Autodesk Inventor part; units mm, degrees
(part 7 of 13)
  arc A2356 (6.9015, 50.997) -> (6.9497, 50.8806) centre (6.9256, 50.9388) ccw
  line L2355 (6.9497, 50.8806) -> (7.4521, 51.0887)
  arc A2357 (7.4521, 51.0887) -> (7.4039, 51.2051) centre (7.428, 51.1469) ccw
  line L2356 (6.8811, 50.9833) -> (6.4966, 50.5988)
  arc A2358 (6.4966, 50.5988) -> (6.5856, 50.5098) centre (6.5411, 50.5543) ccw
  line L2357 (6.5856, 50.5098) -> (6.9701, 50.8943)
  arc A2359 (6.9701, 50.8943) -> (6.8811, 50.9833) centre (6.9256, 50.9388) ccw
  line L2358 (6.4829, 50.5784) -> (6.2748, 50.076)
  arc A2360 (6.2748, 50.076) -> (6.3912, 50.0278) centre (6.333, 50.0519) ccw
  line L2359 (6.3912, 50.0278) -> (6.5993, 50.5302)
  arc A2361 (6.5993, 50.5302) -> (6.4829, 50.5784) centre (6.5411, 50.5543) ccw
  line L2360 (6.27, 50.0519) -> (6.27, 49.8428)
  arc A2362 (6.27, 49.8428) -> (6.396, 49.8428) centre (6.333, 49.8428) ccw
  line L2361 (6.396, 49.8428) -> (6.396, 50.0519)
  arc A2363 (6.396, 50.0519) -> (6.27, 50.0519) centre (6.333, 50.0519) ccw
  line L2362 (6.333, 49.7798) -> (7.6365, 49.7798)
  arc A2364 (7.6365, 49.7798) -> (7.6365, 49.9058) centre (7.6365, 49.8428) ccw
  line L2363 (7.6365, 49.9058) -> (6.333, 49.9058)
  arc A2365 (6.333, 49.9058) -> (6.333, 49.7798) centre (6.333, 49.8428) ccw
  line L2364 (7.5735, 49.8428) -> (7.5735, 49.717)
  arc A2366 (7.5735, 49.717) -> (7.6995, 49.717) centre (7.6365, 49.717) ccw
  line L2365 (7.6995, 49.717) -> (7.6995, 49.8428)
  arc A2367 (7.6995, 49.8428) -> (7.5735, 49.8428) centre (7.6365, 49.8428) ccw
  line L2366 (7.6365, 49.78) -> (6.333, 49.78)
  arc A2368 (6.333, 49.78) -> (6.333, 49.654) centre (6.333, 49.717) ccw
  line L2367 (6.333, 49.654) -> (7.6365, 49.654)
  arc A2369 (7.6365, 49.654) -> (7.6365, 49.78) centre (7.6365, 49.717) ccw
  line L2368 (6.27, 49.717) -> (6.27, 49.508)
  arc A2370 (6.27, 49.508) -> (6.396, 49.508) centre (6.333, 49.508) ccw
  line L2369 (6.396, 49.508) -> (6.396, 49.717)
  arc A2371 (6.396, 49.717) -> (6.27, 49.717) centre (6.333, 49.717) ccw
  line L2370 (6.2748, 49.4839) -> (6.4829, 48.9815)
  arc A2372 (6.4829, 48.9815) -> (6.5993, 49.0297) centre (6.5411, 49.0056) ccw
  line L2371 (6.5993, 49.0297) -> (6.3912, 49.5321)
  arc A2373 (6.3912, 49.5321) -> (6.2748, 49.4839) centre (6.333, 49.508) ccw
  line L2372 (6.4966, 48.9611) -> (6.8811, 48.5766)
  arc A2374 (6.8811, 48.5766) -> (6.9701, 48.6656) centre (6.9256, 48.6211) ccw
  line L2373 (6.9701, 48.6656) -> (6.5856, 49.0501)
  arc A2375 (6.5856, 49.0501) -> (6.4966, 48.9611) centre (6.5411, 49.0056) ccw
  line L2374 (6.9015, 48.5629) -> (7.4039, 48.3548)
  arc A2376 (7.4039, 48.3548) -> (7.4521, 48.4712) centre (7.428, 48.413) ccw
  line L2375 (7.4521, 48.4712) -> (6.9497, 48.6793)
  arc A2377 (6.9497, 48.6793) -> (6.9015, 48.5629) centre (6.9256, 48.6211) ccw
  line L2376 (1.0789, 1.071) -> (17.121, 1.071)
  arc A2378 (17.121, 1.071) -> (17.121, 1.197) centre (17.121, 1.134) ccw
  line L2377 (17.121, 1.197) -> (1.0789, 1.197)
  arc A2379 (1.0789, 1.197) -> (1.0789, 1.071) centre (1.0789, 1.134) ccw
  line L2378 (1.0789, 1.197) -> (17.121, 1.197)
  arc A2380 (17.121, 1.197) -> (17.121, 1.323) centre (17.121, 1.26) ccw
  line L2379 (17.121, 1.323) -> (1.0789, 1.323)
  arc A2381 (1.0789, 1.323) -> (1.0789, 1.197) centre (1.0789, 1.26) ccw
  line L2380 (1.0789, 1.323) -> (17.121, 1.323)
  arc A2382 (17.121, 1.323) -> (17.121, 1.449) centre (17.121, 1.386) ccw
  line L2381 (17.121, 1.449) -> (1.0789, 1.449)
  arc A2383 (1.0789, 1.449) -> (1.0789, 1.323) centre (1.0789, 1.386) ccw
  line L2382 (1.0789, 1.449) -> (17.121, 1.449)
  arc A2384 (17.121, 1.449) -> (17.121, 1.575) centre (17.121, 1.512) ccw
  line L2383 (17.121, 1.575) -> (1.0789, 1.575)
  arc A2385 (1.0789, 1.575) -> (1.0789, 1.449) centre (1.0789, 1.512) ccw
  line L2384 (1.0789, 1.575) -> (17.121, 1.575)
  arc A2386 (17.121, 1.575) -> (17.121, 1.701) centre (17.121, 1.638) ccw
  line L2385 (17.121, 1.701) -> (1.0789, 1.701)
  arc A2387 (1.0789, 1.701) -> (1.0789, 1.575) centre (1.0789, 1.638) ccw
  line L2386 (1.0789, 1.701) -> (17.121, 1.701)
  arc A2388 (17.121, 1.701) -> (17.121, 1.827) centre (17.121, 1.764) ccw
  line L2387 (17.121, 1.827) -> (1.0789, 1.827)
  arc A2389 (1.0789, 1.827) -> (1.0789, 1.701) centre (1.0789, 1.764) ccw
  line L2388 (1.0789, 1.827) -> (17.121, 1.827)
  arc A2390 (17.121, 1.827) -> (17.121, 1.953) centre (17.121, 1.89) ccw
  line L2389 (17.121, 1.953) -> (1.0789, 1.953)
  arc A2391 (1.0789, 1.953) -> (1.0789, 1.827) centre (1.0789, 1.89) ccw
  line L2390 (1.0789, 1.953) -> (17.121, 1.953)
  arc A2392 (17.121, 1.953) -> (17.121, 2.079) centre (17.121, 2.016) ccw
  line L2391 (17.121, 2.079) -> (1.0789, 2.079)
  arc A2393 (1.0789, 2.079) -> (1.0789, 1.953) centre (1.0789, 2.016) ccw
  line L2392 (1.0789, 2.079) -> (17.121, 2.079)
  arc A2394 (17.121, 2.079) -> (17.121, 2.205) centre (17.121, 2.142) ccw
  line L2393 (17.121, 2.205) -> (1.0789, 2.205)
  arc A2395 (1.0789, 2.205) -> (1.0789, 2.079) centre (1.0789, 2.142) ccw
  line L2394 (1.0789, 2.205) -> (17.121, 2.205)
  arc A2396 (17.121, 2.205) -> (17.121, 2.331) centre (17.121, 2.268) ccw
  line L2395 (17.121, 2.331) -> (1.0789, 2.331)
  arc A2397 (1.0789, 2.331) -> (1.0789, 2.205) centre (1.0789, 2.268) ccw
  line L2396 (1.0789, 2.331) -> (17.121, 2.331)
  arc A2398 (17.121, 2.331) -> (17.121, 2.457) centre (17.121, 2.394) ccw
  line L2397 (17.121, 2.457) -> (1.0789, 2.457)
  arc A2399 (1.0789, 2.457) -> (1.0789, 2.331) centre (1.0789, 2.394) ccw
  line L2398 (1.0789, 2.457) -> (17.121, 2.457)
  arc A2400 (17.121, 2.457) -> (17.121, 2.583) centre (17.121, 2.52) ccw
  line L2399 (17.121, 2.583) -> (1.0789, 2.583)
  arc A2401 (1.0789, 2.583) -> (1.0789, 2.457) centre (1.0789, 2.52) ccw
  line L2400 (1.0789, 2.583) -> (17.121, 2.583)
  arc A2402 (17.121, 2.583) -> (17.121, 2.709) centre (17.121, 2.646) ccw
  line L2401 (17.121, 2.709) -> (1.0789, 2.709)
  arc A2403 (1.0789, 2.709) -> (1.0789, 2.583) centre (1.0789, 2.646) ccw
  line L2402 (1.0789, 2.709) -> (17.121, 2.709)
  arc A2404 (17.121, 2.709) -> (17.121, 2.835) centre (17.121, 2.772) ccw
  line L2403 (17.121, 2.835) -> (1.0789, 2.835)
  arc A2405 (1.0789, 2.835) -> (1.0789, 2.709) centre (1.0789, 2.772) ccw
  line L2404 (1.0789, 2.835) -> (6.4573, 2.835)
  arc A2406 (6.4573, 2.835) -> (6.4573, 2.961) centre (6.4573, 2.898) ccw
  line L2405 (6.4573, 2.961) -> (1.0789, 2.961)
  arc A2407 (1.0789, 2.961) -> (1.0789, 2.835) centre (1.0789, 2.898) ccw
  line L2406 (8.9426, 2.835) -> (17.121, 2.835)
  line L2407 (1.0789, 49.833) -> (1.7644, 49.833)
  line L2408 (17.121, 2.961) -> (8.9426, 2.961)
  arc A2408 (8.9426, 2.961) -> (8.9426, 2.835) centre (8.9426, 2.898) ccw
  line L2409 (1.0789, 2.961) -> (6.4346, 2.961)
  arc A2409 (6.4346, 2.961) -> (6.4346, 3.087) centre (6.4346, 3.024) ccw
  line L2410 (6.4346, 3.087) -> (1.0789, 3.087)
  arc A2410 (1.0789, 3.087) -> (1.0789, 2.961) centre (1.0789, 3.024) ccw
  line L2411 (8.9653, 2.961) -> (17.121, 2.961)
  arc A2411 (17.121, 2.961) -> (17.121, 3.087) centre (17.121, 3.024) ccw
  line L2412 (17.121, 3.087) -> (8.9653, 3.087)
  arc A2412 (8.9653, 3.087) -> (8.9653, 2.961) centre (8.9653, 3.024) ccw
  line L2413 (1.0789, 3.087) -> (6.4346, 3.087)
  arc A2413 (6.4346, 3.087) -> (6.4346, 3.213) centre (6.4346, 3.15) ccw
  line L2414 (6.4346, 3.213) -> (1.0789, 3.213)
  arc A2414 (1.0789, 3.213) -> (1.0789, 3.087) centre (1.0789, 3.15) ccw
  line L2415 (8.9653, 3.087) -> (17.121, 3.087)
  arc A2415 (17.121, 3.087) -> (17.121, 3.213) centre (17.121, 3.15) ccw
  line L2416 (17.121, 3.213) -> (8.9653, 3.213)
  arc A2416 (8.9653, 3.213) -> (8.9653, 3.087) centre (8.9653, 3.15) ccw
  line L2417 (1.0789, 3.213) -> (6.4346, 3.213)
  arc A2417 (6.4346, 3.213) -> (6.4346, 3.339) centre (6.4346, 3.276) ccw
  line L2418 (6.4346, 3.339) -> (1.0789, 3.339)
  arc A2418 (1.0789, 3.339) -> (1.0789, 3.213) centre (1.0789, 3.276) ccw
  line L2419 (8.9653, 3.213) -> (17.121, 3.213)
  arc A2419 (17.121, 3.213) -> (17.121, 3.339) centre (17.121, 3.276) ccw
  line L2420 (17.121, 3.339) -> (8.9653, 3.339)
  arc A2420 (8.9653, 3.339) -> (8.9653, 3.213) centre (8.9653, 3.276) ccw
  line L2421 (1.0789, 3.339) -> (6.4346, 3.339)
  arc A2421 (6.4346, 3.339) -> (6.4346, 3.465) centre (6.4346, 3.402) ccw
  line L2422 (6.4346, 3.465) -> (1.0789, 3.465)
  arc A2422 (1.0789, 3.465) -> (1.0789, 3.339) centre (1.0789, 3.402) ccw
  line L2423 (8.9653, 3.339) -> (17.121, 3.339)
  arc A2423 (17.121, 3.339) -> (17.121, 3.465) centre (17.121, 3.402) ccw
  line L2424 (17.121, 3.465) -> (8.9653, 3.465)
  arc A2424 (8.9653, 3.465) -> (8.9653, 3.339) centre (8.9653, 3.402) ccw
  line L2425 (1.0789, 3.465) -> (6.4346, 3.465)
  arc A2425 (6.4346, 3.465) -> (6.4346, 3.591) centre (6.4346, 3.528) ccw
  line L2426 (6.4346, 3.591) -> (1.0789, 3.591)
  arc A2426 (1.0789, 3.591) -> (1.0789, 3.465) centre (1.0789, 3.528) ccw
  line L2427 (8.9653, 3.465) -> (17.121, 3.465)
  arc A2427 (17.121, 3.465) -> (17.121, 3.591) centre (17.121, 3.528) ccw
  line L2428 (17.121, 3.591) -> (8.9653, 3.591)
  arc A2428 (8.9653, 3.591) -> (8.9653, 3.465) centre (8.9653, 3.528) ccw
  line L2429 (1.0789, 3.591) -> (6.4346, 3.591)
  arc A2429 (6.4346, 3.591) -> (6.4346, 3.717) centre (6.4346, 3.654) ccw
  line L2430 (6.4346, 3.717) -> (1.0789, 3.717)
  arc A2430 (1.0789, 3.717) -> (1.0789, 3.591) centre (1.0789, 3.654) ccw
  line L2431 (8.9653, 3.591) -> (17.121, 3.591)
  arc A2431 (17.121, 3.591) -> (17.121, 3.717) centre (17.121, 3.654) ccw
  line L2432 (17.121, 3.717) -> (8.9653, 3.717)
  arc A2432 (8.9653, 3.717) -> (8.9653, 3.591) centre (8.9653, 3.654) ccw
  line L2433 (1.0789, 3.717) -> (6.4346, 3.717)
  arc A2433 (6.4346, 3.717) -> (6.4346, 3.843) centre (6.4346, 3.78) ccw
  line L2434 (6.4346, 3.843) -> (1.0789, 3.843)
  arc A2434 (1.0789, 3.843) -> (1.0789, 3.717) centre (1.0789, 3.78) ccw
  line L2435 (8.9653, 3.717) -> (17.121, 3.717)
  arc A2435 (17.121, 3.717) -> (17.121, 3.843) centre (17.121, 3.78) ccw
  line L2436 (17.121, 3.843) -> (8.9653, 3.843)
  arc A2436 (8.9653, 3.843) -> (8.9653, 3.717) centre (8.9653, 3.78) ccw
  line L2437 (1.0789, 3.843) -> (6.4346, 3.843)
  arc A2437 (6.4346, 3.843) -> (6.4346, 3.969) centre (6.4346, 3.906) ccw
  line L2438 (6.4346, 3.969) -> (1.0789, 3.969)
  arc A2438 (1.0789, 3.969) -> (1.0789, 3.843) centre (1.0789, 3.906) ccw
  line L2439 (8.9653, 3.843) -> (17.121, 3.843)
  arc A2439 (17.121, 3.843) -> (17.121, 3.969) centre (17.121, 3.906) ccw
  line L2440 (17.121, 3.969) -> (8.9653, 3.969)
  arc A2440 (8.9653, 3.969) -> (8.9653, 3.843) centre (8.9653, 3.906) ccw
  line L2441 (1.0789, 3.969) -> (6.4346, 3.969)
  arc A2441 (6.4346, 3.969) -> (6.4346, 4.095) centre (6.4346, 4.032) ccw
  line L2442 (6.4346, 4.095) -> (1.0789, 4.095)
  arc A2442 (1.0789, 4.095) -> (1.0789, 3.969) centre (1.0789, 4.032) ccw
  line L2443 (8.9653, 3.969) -> (17.121, 3.969)
  arc A2443 (17.121, 3.969) -> (17.121, 4.095) centre (17.121, 4.032) ccw
  line L2444 (17.121, 4.095) -> (8.9653, 4.095)
  arc A2444 (8.9653, 4.095) -> (8.9653, 3.969) centre (8.9653, 4.032) ccw
  line L2445 (1.0789, 4.095) -> (6.4346, 4.095)
  arc A2445 (6.4346, 4.095) -> (6.4346, 4.221) centre (6.4346, 4.158) ccw
  line L2446 (6.4346, 4.221) -> (1.0789, 4.221)
  arc A2446 (1.0789, 4.221) -> (1.0789, 4.095) centre (1.0789, 4.158) ccw
  line L2447 (8.9653, 4.095) -> (17.121, 4.095)
  arc A2447 (17.121, 4.095) -> (17.121, 4.221) centre (17.121, 4.158) ccw
  line L2448 (17.121, 4.221) -> (8.9653, 4.221)
  arc A2448 (8.9653, 4.221) -> (8.9653, 4.095) centre (8.9653, 4.158) ccw
  line L2449 (1.0789, 4.221) -> (6.4346, 4.221)
  arc A2449 (6.4346, 4.221) -> (6.4346, 4.347) centre (6.4346, 4.284) ccw
  line L2450 (6.4346, 4.347) -> (1.0789, 4.347)
  arc A2450 (1.0789, 4.347) -> (1.0789, 4.221) centre (1.0789, 4.284) ccw
  line L2451 (8.9653, 4.221) -> (17.121, 4.221)
  arc A2451 (17.121, 4.221) -> (17.121, 4.347) centre (17.121, 4.284) ccw
  line L2452 (17.121, 4.347) -> (8.9653, 4.347)
  arc A2452 (8.9653, 4.347) -> (8.9653, 4.221) centre (8.9653, 4.284) ccw
  line L2453 (1.0789, 4.347) -> (6.4346, 4.347)
  arc A2453 (6.4346, 4.347) -> (6.4346, 4.473) centre (6.4346, 4.41) ccw
  line L2454 (6.4346, 4.473) -> (1.0789, 4.473)
  arc A2454 (1.0789, 4.473) -> (1.0789, 4.347) centre (1.0789, 4.41) ccw
  line L2455 (8.9653, 4.347) -> (17.121, 4.347)
  arc A2455 (17.121, 4.347) -> (17.121, 4.473) centre (17.121, 4.41) ccw
  line L2456 (17.121, 4.473) -> (8.9653, 4.473)
  arc A2456 (8.9653, 4.473) -> (8.9653, 4.347) centre (8.9653, 4.41) ccw
  line L2457 (1.0789, 4.473) -> (6.4346, 4.473)
  arc A2457 (6.4346, 4.473) -> (6.4346, 4.599) centre (6.4346, 4.536) ccw
  line L2458 (6.4346, 4.599) -> (1.0789, 4.599)
  arc A2458 (1.0789, 4.599) -> (1.0789, 4.473) centre (1.0789, 4.536) ccw
  line L2459 (8.9653, 4.473) -> (17.121, 4.473)
  arc A2459 (17.121, 4.473) -> (17.121, 4.599) centre (17.121, 4.536) ccw
  line L2460 (17.121, 4.599) -> (8.9653, 4.599)
  arc A2460 (8.9653, 4.599) -> (8.9653, 4.473) centre (8.9653, 4.536) ccw
  line L2461 (1.0789, 4.599) -> (6.4346, 4.599)
  arc A2461 (6.4346, 4.599) -> (6.4346, 4.725) centre (6.4346, 4.662) ccw
  line L2462 (6.4346, 4.725) -> (1.0789, 4.725)
  arc A2462 (1.0789, 4.725) -> (1.0789, 4.599) centre (1.0789, 4.662) ccw
  line L2463 (8.9653, 4.599) -> (17.121, 4.599)
  arc A2463 (17.121, 4.599) -> (17.121, 4.725) centre (17.121, 4.662) ccw
  line L2464 (17.121, 4.725) -> (8.9653, 4.725)
  arc A2464 (8.9653, 4.725) -> (8.9653, 4.599) centre (8.9653, 4.662) ccw
  line L2465 (1.0789, 4.725) -> (6.4346, 4.725)
  arc A2465 (6.4346, 4.725) -> (6.4346, 4.851) centre (6.4346, 4.788) ccw
  line L2466 (6.4346, 4.851) -> (1.0789, 4.851)
  arc A2466 (1.0789, 4.851) -> (1.0789, 4.725) centre (1.0789, 4.788) ccw
  line L2467 (8.9653, 4.725) -> (17.121, 4.725)
  arc A2467 (17.121, 4.725) -> (17.121, 4.851) centre (17.121, 4.788) ccw
  line L2468 (17.121, 4.851) -> (8.9653, 4.851)
  arc A2468 (8.9653, 4.851) -> (8.9653, 4.725) centre (8.9653, 4.788) ccw
  line L2469 (1.0789, 4.851) -> (6.4346, 4.851)
  arc A2469 (6.4346, 4.851) -> (6.4346, 4.977) centre (6.4346, 4.914) ccw
  line L2470 (6.4346, 4.977) -> (1.0789, 4.977)
  arc A2470 (1.0789, 4.977) -> (1.0789, 4.851) centre (1.0789, 4.914) ccw
  line L2471 (8.9653, 4.851) -> (17.121, 4.851)
  arc A2471 (17.121, 4.851) -> (17.121, 4.977) centre (17.121, 4.914) ccw
  line L2472 (17.121, 4.977) -> (8.9653, 4.977)
  arc A2472 (8.9653, 4.977) -> (8.9653, 4.851) centre (8.9653, 4.914) ccw
  line L2473 (1.0789, 4.977) -> (6.4346, 4.977)
  arc A2473 (6.4346, 4.977) -> (6.4346, 5.103) centre (6.4346, 5.04) ccw
  line L2474 (6.4346, 5.103) -> (1.0789, 5.103)
  arc A2474 (1.0789, 5.103) -> (1.0789, 4.977) centre (1.0789, 5.04) ccw
  line L2475 (8.9653, 4.977) -> (17.121, 4.977)
  arc A2475 (17.121, 4.977) -> (17.121, 5.103) centre (17.121, 5.04) ccw
  line L2476 (17.121, 5.103) -> (8.9653, 5.103)
  arc A2476 (8.9653, 5.103) -> (8.9653, 4.977) centre (8.9653, 5.04) ccw
  line L2477 (1.0789, 5.103) -> (6.4346, 5.103)
  arc A2477 (6.4346, 5.103) -> (6.4346, 5.229) centre (6.4346, 5.166) ccw
  line L2478 (6.4346, 5.229) -> (1.0789, 5.229)
  arc A2478 (1.0789, 5.229) -> (1.0789, 5.103) centre (1.0789, 5.166) ccw
  line L2479 (8.9653, 5.103) -> (17.121, 5.103)
  arc A2479 (17.121, 5.103) -> (17.121, 5.229) centre (17.121, 5.166) ccw
  line L2480 (17.121, 5.229) -> (8.9653, 5.229)
  arc A2480 (8.9653, 5.229) -> (8.9653, 5.103) centre (8.9653, 5.166) ccw
  line L2481 (1.0789, 5.229) -> (6.5274, 5.229)
  arc A2481 (6.5274, 5.229) -> (6.5274, 5.355) centre (6.5274, 5.292) ccw
  line L2482 (6.5274, 5.355) -> (1.0789, 5.355)
  arc A2482 (1.0789, 5.355) -> (1.0789, 5.229) centre (1.0789, 5.292) ccw
  line L2483 (8.8725, 5.229) -> (17.121, 5.229)
  arc A2483 (17.121, 5.229) -> (17.121, 5.355) centre (17.121, 5.292) ccw
  line L2484 (17.121, 5.355) -> (8.8725, 5.355)
  arc A2484 (8.8725, 5.355) -> (8.8725, 5.229) centre (8.8725, 5.292) ccw
  line L2485 (1.0789, 5.355) -> (17.121, 5.355)
  arc A2485 (17.121, 5.355) -> (17.121, 5.481) centre (17.121, 5.418) ccw
  line L2486 (17.121, 5.481) -> (1.0789, 5.481)
  arc A2486 (1.0789, 5.481) -> (1.0789, 5.355) centre (1.0789, 5.418) ccw
  line L2487 (1.0789, 5.481) -> (17.121, 5.481)
  arc A2487 (17.121, 5.481) -> (17.121, 5.607) centre (17.121, 5.544) ccw
  line L2488 (17.121, 5.607) -> (1.0789, 5.607)
  arc A2488 (1.0789, 5.607) -> (1.0789, 5.481) centre (1.0789, 5.544) ccw
  line L2489 (1.0789, 5.607) -> (17.121, 5.607)
  arc A2489 (17.121, 5.607) -> (17.121, 5.733) centre (17.121, 5.67) ccw
  line L2490 (17.121, 5.733) -> (1.0789, 5.733)
  arc A2490 (1.0789, 5.733) -> (1.0789, 5.607) centre (1.0789, 5.67) ccw
  line L2491 (1.0789, 5.733) -> (17.121, 5.733)
  arc A2491 (17.121, 5.733) -> (17.121, 5.859) centre (17.121, 5.796) ccw
  line L2492 (17.121, 5.859) -> (1.0789, 5.859)
  arc A2492 (1.0789, 5.859) -> (1.0789, 5.733) centre (1.0789, 5.796) ccw
  line L2493 (1.0789, 5.859) -> (17.121, 5.859)
  arc A2493 (17.121, 5.859) -> (17.121, 5.985) centre (17.121, 5.922) ccw
  line L2494 (17.121, 5.985) -> (1.0789, 5.985)
  arc A2494 (1.0789, 5.985) -> (1.0789, 5.859) centre (1.0789, 5.922) ccw
  line L2495 (1.0789, 5.985) -> (17.121, 5.985)
  arc A2495 (17.121, 5.985) -> (17.121, 6.111) centre (17.121, 6.048) ccw
  line L2496 (17.121, 6.111) -> (1.0789, 6.111)
  arc A2496 (1.0789, 6.111) -> (1.0789, 5.985) centre (1.0789, 6.048) ccw
  line L2497 (1.0789, 6.111) -> (17.121, 6.111)
  arc A2497 (17.121, 6.111) -> (17.121, 6.237) centre (17.121, 6.174) ccw
  line L2498 (17.121, 6.237) -> (1.0789, 6.237)
  arc A2498 (1.0789, 6.237) -> (1.0789, 6.111) centre (1.0789, 6.174) ccw
  line L2499 (1.0789, 6.237) -> (17.121, 6.237)
  arc A2499 (17.121, 6.237) -> (17.121, 6.363) centre (17.121, 6.3) ccw
  line L2500 (17.121, 6.363) -> (1.0789, 6.363)
  arc A2500 (1.0789, 6.363) -> (1.0789, 6.237) centre (1.0789, 6.3) ccw
  line L2501 (1.0789, 6.363) -> (17.121, 6.363)
  arc A2501 (17.121, 6.363) -> (17.121, 6.489) centre (17.121, 6.426) ccw
  line L2502 (17.121, 6.489) -> (1.0789, 6.489)
  arc A2502 (1.0789, 6.489) -> (1.0789, 6.363) centre (1.0789, 6.426) ccw
  line L2503 (1.0789, 6.489) -> (17.121, 6.489)
  arc A2503 (17.121, 6.489) -> (17.121, 6.615) centre (17.121, 6.552) ccw
  line L2504 (17.121, 6.615) -> (1.0789, 6.615)
  arc A2504 (1.0789, 6.615) -> (1.0789, 6.489) centre (1.0789, 6.552) ccw
  line L2505 (1.0789, 6.615) -> (17.121, 6.615)
  arc A2505 (17.121, 6.615) -> (17.121, 6.741) centre (17.121, 6.678) ccw
  line L2506 (17.121, 6.741) -> (1.0789, 6.741)
  arc A2506 (1.0789, 6.741) -> (1.0789, 6.615) centre (1.0789, 6.678) ccw
  line L2507 (1.0789, 6.741) -> (17.121, 6.741)
  arc A2507 (17.121, 6.741) -> (17.121, 6.867) centre (17.121, 6.804) ccw
  line L2508 (17.121, 6.867) -> (1.0789, 6.867)
  arc A2508 (1.0789, 6.867) -> (1.0789, 6.741) centre (1.0789, 6.804) ccw
  line L2509 (1.0789, 6.867) -> (17.121, 6.867)
  arc A2509 (17.121, 6.867) -> (17.121, 6.993) centre (17.121, 6.93) ccw
  line L2510 (17.121, 6.993) -> (1.0789, 6.993)
  arc A2510 (1.0789, 6.993) -> (1.0789, 6.867) centre (1.0789, 6.93) ccw
  line L2511 (1.0789, 6.993) -> (17.121, 6.993)
  arc A2511 (17.121, 6.993) -> (17.121, 7.119) centre (17.121, 7.056) ccw
  line L2512 (17.121, 7.119) -> (1.0789, 7.119)
  arc A2512 (1.0789, 7.119) -> (1.0789, 6.993) centre (1.0789, 7.056) ccw
  line L2513 (1.0789, 7.119) -> (17.121, 7.119)
  arc A2513 (17.121, 7.119) -> (17.121, 7.245) centre (17.121, 7.182) ccw
  line L2514 (17.121, 7.245) -> (1.0789, 7.245)
  arc A2514 (1.0789, 7.245) -> (1.0789, 7.119) centre (1.0789, 7.182) ccw
  line L2515 (1.0789, 7.245) -> (17.121, 7.245)
  arc A2515 (17.121, 7.245) -> (17.121, 7.371) centre (17.121, 7.308) ccw
  line L2516 (17.121, 7.371) -> (1.0789, 7.371)
  arc A2516 (1.0789, 7.371) -> (1.0789, 7.245) centre (1.0789, 7.308) ccw
  line L2517 (1.0789, 7.371) -> (17.121, 7.371)
  arc A2517 (17.121, 7.371) -> (17.121, 7.497) centre (17.121, 7.434) ccw
  line L2518 (17.121, 7.497) -> (1.0789, 7.497)
  arc A2518 (1.0789, 7.497) -> (1.0789, 7.371) centre (1.0789, 7.434) ccw
  line L2519 (1.0789, 7.497) -> (17.121, 7.497)
  arc A2519 (17.121, 7.497) -> (17.121, 7.623) centre (17.121, 7.56) ccw
  line L2520 (17.121, 7.623) -> (1.0789, 7.623)
  arc A2520 (1.0789, 7.623) -> (1.0789, 7.497) centre (1.0789, 7.56) ccw
  line L2521 (1.0789, 7.623) -> (17.121, 7.623)
  arc A2521 (17.121, 7.623) -> (17.121, 7.749) centre (17.121, 7.686) ccw
  line L2522 (17.121, 7.749) -> (1.0789, 7.749)
  arc A2522 (1.0789, 7.749) -> (1.0789, 7.623) centre (1.0789, 7.686) ccw
  line L2523 (1.0789, 7.749) -> (7.3338, 7.749)
  arc A2523 (7.3338, 7.749) -> (7.3338, 7.875) centre (7.3338, 7.812) ccw
  line L2524 (7.3338, 7.875) -> (1.0789, 7.875)
  arc A2524 (1.0789, 7.875) -> (1.0789, 7.749) centre (1.0789, 7.812) ccw
  line L2525 (7.637, 7.749) -> (7.7628, 7.749)
  arc A2525 (7.7628, 7.749) -> (7.7628, 7.875) centre (7.7628, 7.812) ccw
  line L2526 (7.7628, 7.875) -> (7.637, 7.875)
  arc A2526 (7.637, 7.875) -> (7.637, 7.749) centre (7.637, 7.812) ccw
  line L2527 (8.066, 7.749) -> (17.121, 7.749)
  arc A2527 (17.121, 7.749) -> (17.121, 7.875) centre (17.121, 7.812) ccw
  line L2528 (17.121, 7.875) -> (8.066, 7.875)
  arc A2528 (8.066, 7.875) -> (8.066, 7.749) centre (8.066, 7.812) ccw
  line L2529 (1.0789, 7.875) -> (7.0296, 7.875)
  arc A2529 (7.0296, 7.875) -> (7.0296, 8.001) centre (7.0296, 7.938) ccw
  line L2530 (7.0296, 8.001) -> (1.0789, 8.001)
  arc A2530 (1.0789, 8.001) -> (1.0789, 7.875) centre (1.0789, 7.938) ccw
  line L2531 (7.637, 7.875) -> (7.7628, 7.875)
  arc A2531 (7.7628, 7.875) -> (7.7628, 8.001) centre (7.7628, 7.938) ccw
  line L2532 (7.7628, 8.001) -> (7.637, 8.001)
  arc A2532 (7.637, 8.001) -> (7.637, 7.875) centre (7.637, 7.938) ccw
  line L2533 (8.3702, 7.875) -> (17.121, 7.875)
  arc A2533 (17.121, 7.875) -> (17.121, 8.001) centre (17.121, 7.938) ccw
  line L2534 (17.121, 8.001) -> (8.3702, 8.001)
  arc A2534 (8.3702, 8.001) -> (8.3702, 7.875) centre (8.3702, 7.938) ccw
  line L2535 (1.0789, 8.001) -> (6.8427, 8.001)
  arc A2535 (6.8427, 8.001) -> (6.8427, 8.127) centre (6.8427, 8.064) ccw
  line L2536 (6.8427, 8.127) -> (1.0789, 8.127)
  arc A2536 (1.0789, 8.127) -> (1.0789, 8.001) centre (1.0789, 8.064) ccw
  line L2537 (7.637, 8.001) -> (7.7628, 8.001)
  arc A2537 (7.7628, 8.001) -> (7.7628, 8.127) centre (7.7628, 8.064) ccw
  line L2538 (7.7628, 8.127) -> (7.637, 8.127)
  arc A2538 (7.637, 8.127) -> (7.637, 8.001) centre (7.637, 8.064) ccw
  line L2539 (8.5572, 8.001) -> (17.121, 8.001)
  arc A2539 (17.121, 8.001) -> (17.121, 8.127) centre (17.121, 8.064) ccw
  line L2540 (17.121, 8.127) -> (8.5572, 8.127)
  arc A2540 (8.5572, 8.127) -> (8.5572, 8.001) centre (8.5572, 8.064) ccw
  line L2541 (1.0789, 8.127) -> (6.7167, 8.127)
  arc A2541 (6.7167, 8.127) -> (6.7167, 8.253) centre (6.7167, 8.19) ccw
  line L2542 (6.7167, 8.253) -> (1.0789, 8.253)
  arc A2542 (1.0789, 8.253) -> (1.0789, 8.127) centre (1.0789, 8.19) ccw
  line L2543 (7.637, 8.127) -> (7.7628, 8.127)
  arc A2543 (7.7628, 8.127) -> (7.7628, 8.253) centre (7.7628, 8.19) ccw
  line L2544 (7.7628, 8.253) -> (7.637, 8.253)
  arc A2544 (7.637, 8.253) -> (7.637, 8.127) centre (7.637, 8.19) ccw
  line L2545 (8.6832, 8.127) -> (17.121, 8.127)
  arc A2545 (17.121, 8.127) -> (17.121, 8.253) centre (17.121, 8.19) ccw
  line L2546 (17.121, 8.253) -> (8.6832, 8.253)
  arc A2546 (8.6832, 8.253) -> (8.6832, 8.127) centre (8.6832, 8.19) ccw
  line L2547 (1.0789, 8.253) -> (6.5907, 8.253)
  arc A2547 (6.5907, 8.253) -> (6.5907, 8.379) centre (6.5907, 8.316) ccw
  line L2548 (6.5907, 8.379) -> (1.0789, 8.379)
  arc A2548 (1.0789, 8.379) -> (1.0789, 8.253) centre (1.0789, 8.316) ccw
  line L2549 (7.637, 8.253) -> (7.7628, 8.253)
  arc A2549 (7.7628, 8.253) -> (7.7628, 8.379) centre (7.7628, 8.316) ccw
  line L2550 (7.7628, 8.379) -> (7.637, 8.379)
  arc A2550 (7.637, 8.379) -> (7.637, 8.253) centre (7.637, 8.316) ccw
  line L2551 (8.8092, 8.253) -> (17.121, 8.253)
  arc A2551 (17.121, 8.253) -> (17.121, 8.379) centre (17.121, 8.316) ccw
  line L2552 (17.121, 8.379) -> (8.8092, 8.379)
  arc A2552 (8.8092, 8.379) -> (8.8092, 8.253) centre (8.8092, 8.316) ccw
  line L2553 (1.0789, 8.379) -> (6.5094, 8.379)
  arc A2553 (6.5094, 8.379) -> (6.5094, 8.505) centre (6.5094, 8.442) ccw
  line L2554 (6.5094, 8.505) -> (1.0789, 8.505)
  arc A2554 (1.0789, 8.505) -> (1.0789, 8.379) centre (1.0789, 8.442) ccw
  line L2555 (7.637, 8.379) -> (7.7628, 8.379)
  arc A2555 (7.7628, 8.379) -> (7.7628, 8.505) centre (7.7628, 8.442) ccw
  line L2556 (7.7628, 8.505) -> (7.637, 8.505)
  arc A2556 (7.637, 8.505) -> (7.637, 8.379) centre (7.637, 8.442) ccw
  line L2557 (8.8904, 8.379) -> (17.121, 8.379)
  arc A2557 (17.121, 8.379) -> (17.121, 8.505) centre (17.121, 8.442) ccw
  line L2558 (17.121, 8.505) -> (8.8904, 8.505)
  arc A2558 (8.8904, 8.505) -> (8.8904, 8.379) centre (8.8904, 8.442) ccw
  line L2559 (1.0789, 8.505) -> (6.4572, 8.505)
  arc A2559 (6.4572, 8.505) -> (6.4572, 8.631) centre (6.4572, 8.568) ccw
  line L2560 (6.4572, 8.631) -> (1.0789, 8.631)
  arc A2560 (1.0789, 8.631) -> (1.0789, 8.505) centre (1.0789, 8.568) ccw
  line L2561 (7.637, 8.505) -> (7.7628, 8.505)
  arc A2561 (7.7628, 8.505) -> (7.7628, 8.631) centre (7.7628, 8.568) ccw
  line L2562 (7.7628, 8.631) -> (7.637, 8.631)
  arc A2562 (7.637, 8.631) -> (7.637, 8.505) centre (7.637, 8.568) ccw
  line L2563 (8.9426, 8.505) -> (17.121, 8.505)
  arc A2563 (17.121, 8.505) -> (17.121, 8.631) centre (17.121, 8.568) ccw
  line L2564 (17.121, 8.631) -> (8.9426, 8.631)
  arc A2564 (8.9426, 8.631) -> (8.9426, 8.505) centre (8.9426, 8.568) ccw
  line L2565 (1.0789, 8.631) -> (6.405, 8.631)
  arc A2565 (6.405, 8.631) -> (6.405, 8.757) centre (6.405, 8.694) ccw
  line L2566 (6.405, 8.757) -> (1.0789, 8.757)
  arc A2566 (1.0789, 8.757) -> (1.0789, 8.631) centre (1.0789, 8.694) ccw
  line L2567 (7.637, 8.631) -> (7.7628, 8.631)
  arc A2567 (7.7628, 8.631) -> (7.7628, 8.757) centre (7.7628, 8.694) ccw
  line L2568 (7.7628, 8.757) -> (7.637, 8.757)
  arc A2568 (7.637, 8.757) -> (7.637, 8.631) centre (7.637, 8.694) ccw
  line L2569 (8.9948, 8.631) -> (17.121, 8.631)
  arc A2569 (17.121, 8.631) -> (17.121, 8.757) centre (17.121, 8.694) ccw
  line L2570 (17.121, 8.757) -> (8.9948, 8.757)
  arc A2570 (8.9948, 8.757) -> (8.9948, 8.631) centre (8.9948, 8.694) ccw
  line L2571 (1.0789, 8.757) -> (6.3528, 8.757)
  arc A2571 (6.3528, 8.757) -> (6.3528, 8.883) centre (6.3528, 8.82) ccw
  line L2572 (6.3528, 8.883) -> (1.0789, 8.883)
  arc A2572 (1.0789, 8.883) -> (1.0789, 8.757) centre (1.0789, 8.82) ccw
  line L2573 (7.637, 8.757) -> (7.7628, 8.757)
  arc A2573 (7.7628, 8.757) -> (7.7628, 8.883) centre (7.7628, 8.82) ccw
  line L2574 (7.7628, 8.883) -> (7.637, 8.883)
  arc A2574 (7.637, 8.883) -> (7.637, 8.757) centre (7.637, 8.82) ccw
  line L2575 (9.047, 8.757) -> (17.121, 8.757)
  arc A2575 (17.121, 8.757) -> (17.121, 8.883) centre (17.121, 8.82) ccw
  line L2576 (17.121, 8.883) -> (9.047, 8.883)
  arc A2576 (9.047, 8.883) -> (9.047, 8.757) centre (9.047, 8.82) ccw
  line L2577 (1.0789, 8.883) -> (6.333, 8.883)
  arc A2577 (6.333, 8.883) -> (6.333, 9.009) centre (6.333, 8.946) ccw
  line L2578 (6.333, 9.009) -> (1.0789, 9.009)
  arc A2578 (1.0789, 9.009) -> (1.0789, 8.883) centre (1.0789, 8.946) ccw
  line L2579 (7.637, 8.883) -> (7.7628, 8.883)
  arc A2579 (7.7628, 8.883) -> (7.7628, 9.009) centre (7.7628, 8.946) ccw
  line L2580 (7.7628, 9.009) -> (7.637, 9.009)
  arc A2580 (7.637, 9.009) -> (7.637, 8.883) centre (7.637, 8.946) ccw
  line L2581 (9.0669, 8.883) -> (17.121, 8.883)
  arc A2581 (17.121, 8.883) -> (17.121, 9.009) centre (17.121, 8.946) ccw
  line L2582 (17.121, 9.009) -> (9.0669, 9.009)
  arc A2582 (9.0669, 9.009) -> (9.0669, 8.883) centre (9.0669, 8.946) ccw
  line L2583 (1.0789, 9.009) -> (6.333, 9.009)
  arc A2583 (6.333, 9.009) -> (6.333, 9.135) centre (6.333, 9.072) ccw
  line L2584 (6.333, 9.135) -> (1.0789, 9.135)
  arc A2584 (1.0789, 9.135) -> (1.0789, 9.009) centre (1.0789, 9.072) ccw
  line L2585 (7.637, 9.009) -> (7.7628, 9.009)
  arc A2585 (7.7628, 9.009) -> (7.7628, 9.135) centre (7.7628, 9.072) ccw
  line L2586 (7.7628, 9.135) -> (7.637, 9.135)
  arc A2586 (7.637, 9.135) -> (7.637, 9.009) centre (7.637, 9.072) ccw
  line L2587 (9.0669, 9.009) -> (17.121, 9.009)
  arc A2587 (17.121, 9.009) -> (17.121, 9.135) centre (17.121, 9.072) ccw
  line L2588 (17.121, 9.135) -> (9.0669, 9.135)
  arc A2588 (9.0669, 9.135) -> (9.0669, 9.009) centre (9.0669, 9.072) ccw
  line L2589 (1.0789, 9.135) -> (7.6365, 9.135)
  arc A2589 (7.6365, 9.135) -> (7.6365, 9.261) centre (7.6365, 9.198) ccw
  line L2590 (7.6365, 9.261) -> (1.0789, 9.261)
  arc A2590 (1.0789, 9.261) -> (1.0789, 9.135) centre (1.0789, 9.198) ccw
  line L2591 (7.7634, 9.135) -> (17.121, 9.135)
  arc A2591 (17.121, 9.135) -> (17.121, 9.261) centre (17.121, 9.198) ccw
  line L2592 (17.121, 9.261) -> (7.7634, 9.261)
  arc A2592 (7.7634, 9.261) -> (7.7634, 9.135) centre (7.7634, 9.198) ccw
  line L2593 (1.0789, 9.261) -> (6.333, 9.261)
  arc A2593 (6.333, 9.261) -> (6.333, 9.387) centre (6.333, 9.324) ccw
  line L2594 (6.333, 9.387) -> (1.0789, 9.387)
  arc A2594 (1.0789, 9.387) -> (1.0789, 9.261) centre (1.0789, 9.324) ccw
  line L2595 (7.637, 9.261) -> (7.7628, 9.261)
  arc A2595 (7.7628, 9.261) -> (7.7628, 9.387) centre (7.7628, 9.324) ccw
  line L2596 (7.7628, 9.387) -> (7.637, 9.387)
  arc A2596 (7.637, 9.387) -> (7.637, 9.261) centre (7.637, 9.324) ccw
  line L2597 (9.0669, 9.261) -> (17.121, 9.261)
  arc A2597 (17.121, 9.261) -> (17.121, 9.387) centre (17.121, 9.324) ccw
  line L2598 (17.121, 9.387) -> (9.0669, 9.387)
  arc A2598 (9.0669, 9.387) -> (9.0669, 9.261) centre (9.0669, 9.324) ccw
  line L2599 (1.0789, 9.387) -> (6.3488, 9.387)
  arc A2599 (6.3488, 9.387) -> (6.3488, 9.513) centre (6.3488, 9.45) ccw
  line L2600 (6.3488, 9.513) -> (1.0789, 9.513)
  arc A2600 (1.0789, 9.513) -> (1.0789, 9.387) centre (1.0789, 9.45) ccw
  line L2601 (7.637, 9.387) -> (7.7628, 9.387)
  arc A2601 (7.7628, 9.387) -> (7.7628, 9.513) centre (7.7628, 9.45) ccw
  line L2602 (7.7628, 9.513) -> (7.637, 9.513)
  arc A2602 (7.637, 9.513) -> (7.637, 9.387) centre (7.637, 9.45) ccw
  line L2603 (9.0512, 9.387) -> (17.121, 9.387)
  arc A2603 (17.121, 9.387) -> (17.121, 9.513) centre (17.121, 9.45) ccw
  line L2604 (17.121, 9.513) -> (9.0512, 9.513)
  arc A2604 (9.0512, 9.513) -> (9.0512, 9.387) centre (9.0512, 9.45) ccw
  line L2605 (1.0789, 9.513) -> (6.401, 9.513)
  arc A2605 (6.401, 9.513) -> (6.401, 9.639) centre (6.401, 9.576) ccw
  line L2606 (6.401, 9.639) -> (1.0789, 9.639)
  arc A2606 (1.0789, 9.639) -> (1.0789, 9.513) centre (1.0789, 9.576) ccw
  line L2607 (7.637, 9.513) -> (7.7628, 9.513)
  arc A2607 (7.7628, 9.513) -> (7.7628, 9.639) centre (7.7628, 9.576) ccw
  line L2608 (7.7628, 9.639) -> (7.637, 9.639)
  arc A2608 (7.637, 9.639) -> (7.637, 9.513) centre (7.637, 9.576) ccw
  line L2609 (8.999, 9.513) -> (17.121, 9.513)
  arc A2609 (17.121, 9.513) -> (17.121, 9.639) centre (17.121, 9.576) ccw
  line L2610 (17.121, 9.639) -> (8.999, 9.639)
  arc A2610 (8.999, 9.639) -> (8.999, 9.513) centre (8.999, 9.576) ccw
  line L2611 (1.0789, 9.639) -> (6.4532, 9.639)
  arc A2611 (6.4532, 9.639) -> (6.4532, 9.765) centre (6.4532, 9.702) ccw
  line L2612 (6.4532, 9.765) -> (1.0789, 9.765)
  arc A2612 (1.0789, 9.765) -> (1.0789, 9.639) centre (1.0789, 9.702) ccw
  line L2613 (7.637, 9.639) -> (7.7628, 9.639)
  arc A2613 (7.7628, 9.639) -> (7.7628, 9.765) centre (7.7628, 9.702) ccw
  line L2614 (7.7628, 9.765) -> (7.637, 9.765)
  arc A2614 (7.637, 9.765) -> (7.637, 9.639) centre (7.637, 9.702) ccw
  line L2615 (8.9468, 9.639) -> (17.121, 9.639)
  arc A2615 (17.121, 9.639) -> (17.121, 9.765) centre (17.121, 9.702) ccw
  line L2616 (17.121, 9.765) -> (8.9468, 9.765)
  arc A2616 (8.9468, 9.765) -> (8.9468, 9.639) centre (8.9468, 9.702) ccw
  line L2617 (1.0789, 9.765) -> (6.5054, 9.765)
  arc A2617 (6.5054, 9.765) -> (6.5054, 9.891) centre (6.5054, 9.828) ccw
  line L2618 (6.5054, 9.891) -> (1.0789, 9.891)
  arc A2618 (1.0789, 9.891) -> (1.0789, 9.765) centre (1.0789, 9.828) ccw
  line L2619 (7.637, 9.765) -> (7.7628, 9.765)
  arc A2619 (7.7628, 9.765) -> (7.7628, 9.891) centre (7.7628, 9.828) ccw
  line L2620 (7.7628, 9.891) -> (7.637, 9.891)
  arc A2620 (7.637, 9.891) -> (7.637, 9.765) centre (7.637, 9.828) ccw
  line L2621 (8.8946, 9.765) -> (17.121, 9.765)
  arc A2621 (17.121, 9.765) -> (17.121, 9.891) centre (17.121, 9.828) ccw
  line L2622 (17.121, 9.891) -> (8.8946, 9.891)
  arc A2622 (8.8946, 9.891) -> (8.8946, 9.765) centre (8.8946, 9.828) ccw
  line L2623 (1.0789, 9.891) -> (6.5808, 9.891)
  arc A2623 (6.5808, 9.891) -> (6.5808, 10.017) centre (6.5808, 9.954) ccw
  line L2624 (6.5808, 10.017) -> (1.0789, 10.017)
  arc A2624 (1.0789, 10.017) -> (1.0789, 9.891) centre (1.0789, 9.954) ccw
  line L2625 (7.637, 9.891) -> (7.7628, 9.891)
  arc A2625 (7.7628, 9.891) -> (7.7628, 10.017) centre (7.7628, 9.954) ccw
  line L2626 (7.7628, 10.017) -> (7.637, 10.017)
  arc A2626 (7.637, 10.017) -> (7.637, 9.891) centre (7.637, 9.954) ccw
  line L2627 (8.8191, 9.891) -> (17.121, 9.891)
  arc A2627 (17.121, 9.891) -> (17.121, 10.017) centre (17.121, 9.954) ccw
  line L2628 (17.121, 10.017) -> (8.8191, 10.017)
  arc A2628 (8.8191, 10.017) -> (8.8191, 9.891) centre (8.8191, 9.954) ccw
  line L2629 (1.0789, 10.017) -> (6.7068, 10.017)
  arc A2629 (6.7068, 10.017) -> (6.7068, 10.143) centre (6.7068, 10.08) ccw
  line L2630 (6.7068, 10.143) -> (1.0789, 10.143)
  arc A2630 (1.0789, 10.143) -> (1.0789, 10.017) centre (1.0789, 10.08) ccw
  line L2631 (7.637, 10.017) -> (7.7628, 10.017)
  arc A2631 (7.7628, 10.017) -> (7.7628, 10.143) centre (7.7628, 10.08) ccw
  line L2632 (7.7628, 10.143) -> (7.637, 10.143)
  arc A2632 (7.637, 10.143) -> (7.637, 10.017) centre (7.637, 10.08) ccw
  line L2633 (8.6931, 10.017) -> (17.121, 10.017)
  arc A2633 (17.121, 10.017) -> (17.121, 10.143) centre (17.121, 10.08) ccw
  line L2634 (17.121, 10.143) -> (8.6931, 10.143)
  arc A2634 (8.6931, 10.143) -> (8.6931, 10.017) centre (8.6931, 10.08) ccw
  line L2635 (1.0789, 10.143) -> (6.8328, 10.143)
  arc A2635 (6.8328, 10.143) -> (6.8328, 10.269) centre (6.8328, 10.206) ccw
  line L2636 (6.8328, 10.269) -> (1.0789, 10.269)
  arc A2636 (1.0789, 10.269) -> (1.0789, 10.143) centre (1.0789, 10.206) ccw
  line L2637 (7.637, 10.143) -> (7.7628, 10.143)
  arc A2637 (7.7628, 10.143) -> (7.7628, 10.269) centre (7.7628, 10.206) ccw
  line L2638 (7.7628, 10.269) -> (7.637, 10.269)
  arc A2638 (7.637, 10.269) -> (7.637, 10.143) centre (7.637, 10.206) ccw
  line L2639 (8.5671, 10.143) -> (17.121, 10.143)
  arc A2639 (17.121, 10.143) -> (17.121, 10.269) centre (17.121, 10.206) ccw
  line L2640 (17.121, 10.269) -> (8.5671, 10.269)
  arc A2640 (8.5671, 10.269) -> (8.5671, 10.143) centre (8.5671, 10.206) ccw
  line L2641 (1.0789, 10.269) -> (7.0058, 10.269)
  arc A2641 (7.0058, 10.269) -> (7.0058, 10.395) centre (7.0058, 10.332) ccw
  line L2642 (7.0058, 10.395) -> (1.0789, 10.395)
  arc A2642 (1.0789, 10.395) -> (1.0789, 10.269) centre (1.0789, 10.332) ccw
  line L2643 (7.637, 10.269) -> (7.7628, 10.269)
  arc A2643 (7.7628, 10.269) -> (7.7628, 10.395) centre (7.7628, 10.332) ccw
  line L2644 (7.7628, 10.395) -> (7.637, 10.395)
  arc A2644 (7.637, 10.395) -> (7.637, 10.269) centre (7.637, 10.332) ccw
  line L2645 (8.3942, 10.269) -> (17.121, 10.269)
  arc A2645 (17.121, 10.269) -> (17.121, 10.395) centre (17.121, 10.332) ccw
  line L2646 (17.121, 10.395) -> (8.3942, 10.395)
  arc A2646 (8.3942, 10.395) -> (8.3942, 10.269) centre (8.3942, 10.332) ccw
  line L2647 (1.0789, 10.395) -> (7.31, 10.395)
  arc A2647 (7.31, 10.395) -> (7.31, 10.521) centre (7.31, 10.458) ccw
  line L2648 (7.31, 10.521) -> (1.0789, 10.521)
  arc A2648 (1.0789, 10.521) -> (1.0789, 10.395) centre (1.0789, 10.458) ccw
  line L2649 (7.637, 10.395) -> (7.7628, 10.395)
  arc A2649 (7.7628, 10.395) -> (7.7628, 10.521) centre (7.7628, 10.458) ccw
  line L2650 (7.7628, 10.521) -> (7.637, 10.521)
  arc A2650 (7.637, 10.521) -> (7.637, 10.395) centre (7.637, 10.458) ccw
  line L2651 (8.09, 10.395) -> (17.121, 10.395)
  arc A2651 (17.121, 10.395) -> (17.121, 10.521) centre (17.121, 10.458) ccw
  line L2652 (17.121, 10.521) -> (8.09, 10.521)
  arc A2652 (8.09, 10.521) -> (8.09, 10.395) centre (8.09, 10.458) ccw
  line L2653 (1.0789, 10.521) -> (17.121, 10.521)
  arc A2653 (17.121, 10.521) -> (17.121, 10.647) centre (17.121, 10.584) ccw
  line L2654 (17.121, 10.647) -> (1.0789, 10.647)
  arc A2654 (1.0789, 10.647) -> (1.0789, 10.521) centre (1.0789, 10.584) ccw
  line L2655 (1.0789, 10.647) -> (17.121, 10.647)
  arc A2655 (17.121, 10.647) -> (17.121, 10.773) centre (17.121, 10.71) ccw
  line L2656 (17.121, 10.773) -> (1.0789, 10.773)
  arc A2656 (1.0789, 10.773) -> (1.0789, 10.647) centre (1.0789, 10.71) ccw
  line L2657 (1.0789, 10.773) -> (17.121, 10.773)
  arc A2657 (17.121, 10.773) -> (17.121, 10.899) centre (17.121, 10.836) ccw
  line L2658 (17.121, 10.899) -> (1.0789, 10.899)
  arc A2658 (1.0789, 10.899) -> (1.0789, 10.773) centre (1.0789, 10.836) ccw
  line L2659 (1.0789, 10.899) -> (17.121, 10.899)
  arc A2659 (17.121, 10.899) -> (17.121, 11.025) centre (17.121, 10.962) ccw
  line L2660 (17.121, 11.025) -> (1.0789, 11.025)
  arc A2660 (1.0789, 11.025) -> (1.0789, 10.899) centre (1.0789, 10.962) ccw
  line L2661 (1.0789, 11.025) -> (17.121, 11.025)
  arc A2661 (17.121, 11.025) -> (17.121, 11.151) centre (17.121, 11.088) ccw
  line L2662 (17.121, 11.151) -> (1.0789, 11.151)
  arc A2662 (1.0789, 11.151) -> (1.0789, 11.025) centre (1.0789, 11.088) ccw
  line L2663 (1.0789, 11.151) -> (17.121, 11.151)
  arc A2663 (17.121, 11.151) -> (17.121, 11.277) centre (17.121, 11.214) ccw
  line L2664 (17.121, 11.277) -> (1.0789, 11.277)
  arc A2664 (1.0789, 11.277) -> (1.0789, 11.151) centre (1.0789, 11.214) ccw
  line L2665 (1.0789, 11.277) -> (17.121, 11.277)
  arc A2665 (17.121, 11.277) -> (17.121, 11.403) centre (17.121, 11.34) ccw
  line L2666 (17.121, 11.403) -> (1.0789, 11.403)
  arc A2666 (1.0789, 11.403) -> (1.0789, 11.277) centre (1.0789, 11.34) ccw
  line L2667 (1.0789, 11.403) -> (17.121, 11.403)
  arc A2667 (17.121, 11.403) -> (17.121, 11.529) centre (17.121, 11.466) ccw
  line L2668 (17.121, 11.529) -> (1.0789, 11.529)
  arc A2668 (1.0789, 11.529) -> (1.0789, 11.403) centre (1.0789, 11.466) ccw
  line L2669 (1.0789, 11.529) -> (17.121, 11.529)
  arc A2669 (17.121, 11.529) -> (17.121, 11.655) centre (17.121, 11.592) ccw
  line L2670 (17.121, 11.655) -> (1.0789, 11.655)
  arc A2670 (1.0789, 11.655) -> (1.0789, 11.529) centre (1.0789, 11.592) ccw
  line L2671 (1.0789, 11.655) -> (17.121, 11.655)
  arc A2671 (17.121, 11.655) -> (17.121, 11.781) centre (17.121, 11.718) ccw
  line L2672 (17.121, 11.781) -> (1.0789, 11.781)
  arc A2672 (1.0789, 11.781) -> (1.0789, 11.655) centre (1.0789, 11.718) ccw
  line L2673 (1.0789, 11.781) -> (17.121, 11.781)
  arc A2673 (17.121, 11.781) -> (17.121, 11.907) centre (17.121, 11.844) ccw
  line L2674 (17.121, 11.907) -> (1.0789, 11.907)
  arc A2674 (1.0789, 11.907) -> (1.0789, 11.781) centre (1.0789, 11.844) ccw
  line L2675 (1.0789, 11.907) -> (17.121, 11.907)
  arc A2675 (17.121, 11.907) -> (17.121, 12.033) centre (17.121, 11.97) ccw
  line L2676 (17.121, 12.033) -> (1.0789, 12.033)
  arc A2676 (1.0789, 12.033) -> (1.0789, 11.907) centre (1.0789, 11.97) ccw
  line L2677 (1.0789, 12.033) -> (17.121, 12.033)
  arc A2677 (17.121, 12.033) -> (17.121, 12.159) centre (17.121, 12.096) ccw
  line L2678 (17.121, 12.159) -> (1.0789, 12.159)
  arc A2678 (1.0789, 12.159) -> (1.0789, 12.033) centre (1.0789, 12.096) ccw
  line L2679 (1.0789, 12.159) -> (17.121, 12.159)
  arc A2679 (17.121, 12.159) -> (17.121, 12.285) centre (17.121, 12.222) ccw
  line L2680 (17.121, 12.285) -> (1.0789, 12.285)
  arc A2680 (1.0789, 12.285) -> (1.0789, 12.159) centre (1.0789, 12.222) ccw
  line L2681 (1.0789, 12.285) -> (17.121, 12.285)
  arc A2681 (17.121, 12.285) -> (17.121, 12.411) centre (17.121, 12.348) ccw
  line L2682 (17.121, 12.411) -> (1.0789, 12.411)
  arc A2682 (1.0789, 12.411) -> (1.0789, 12.285) centre (1.0789, 12.348) ccw
  line L2683 (1.0789, 12.411) -> (17.121, 12.411)
  arc A2683 (17.121, 12.411) -> (17.121, 12.537) centre (17.121, 12.474) ccw
  line L2684 (17.121, 12.537) -> (1.0789, 12.537)
  arc A2684 (1.0789, 12.537) -> (1.0789, 12.411) centre (1.0789, 12.474) ccw
  line L2685 (1.0789, 12.537) -> (17.121, 12.537)
  arc A2685 (17.121, 12.537) -> (17.121, 12.663) centre (17.121, 12.6) ccw
  line L2686 (17.121, 12.663) -> (1.0789, 12.663)
  arc A2686 (1.0789, 12.663) -> (1.0789, 12.537) centre (1.0789, 12.6) ccw
  line L2687 (1.0789, 12.663) -> (17.121, 12.663)
  arc A2687 (17.121, 12.663) -> (17.121, 12.789) centre (17.121, 12.726) ccw
  line L2688 (17.121, 12.789) -> (1.0789, 12.789)
  arc A2688 (1.0789, 12.789) -> (1.0789, 12.663) centre (1.0789, 12.726) ccw
  line L2689 (1.0789, 12.789) -> (17.121, 12.789)
  arc A2689 (17.121, 12.789) -> (17.121, 12.915) centre (17.121, 12.852) ccw
  line L2690 (17.121, 12.915) -> (1.0789, 12.915)
  arc A2690 (1.0789, 12.915) -> (1.0789, 12.789) centre (1.0789, 12.852) ccw
  line L2691 (1.0789, 12.915) -> (7.3917, 12.915)
  arc A2691 (7.3917, 12.915) -> (7.3917, 13.041) centre (7.3917, 12.978) ccw
  line L2692 (7.3917, 13.041) -> (1.0789, 13.041)
  arc A2692 (1.0789, 13.041) -> (1.0789, 12.915) centre (1.0789, 12.978) ccw
  line L2693 (8.0081, 12.915) -> (17.121, 12.915)
  arc A2693 (17.121, 12.915) -> (17.121, 13.041) centre (17.121, 12.978) ccw
  line L2694 (17.121, 13.041) -> (8.0081, 13.041)
  arc A2694 (8.0081, 13.041) -> (8.0081, 12.915) centre (8.0081, 12.978) ccw
  line L2695 (1.0789, 13.041) -> (7.0874, 13.041)
  arc A2695 (7.0874, 13.041) -> (7.0874, 13.167) centre (7.0874, 13.104) ccw
  line L2696 (7.0874, 13.167) -> (1.0789, 13.167)
  arc A2696 (1.0789, 13.167) -> (1.0789, 13.041) centre (1.0789, 13.104) ccw
  line L2697 (8.3124, 13.041) -> (17.121, 13.041)
  arc A2697 (17.121, 13.041) -> (17.121, 13.167) centre (17.121, 13.104) ccw
  line L2698 (17.121, 13.167) -> (8.3124, 13.167)
  arc A2698 (8.3124, 13.167) -> (8.3124, 13.041) centre (8.3124, 13.104) ccw
  line L2699 (1.0789, 13.167) -> (6.9004, 13.167)
  arc A2699 (6.9004, 13.167) -> (6.9004, 13.293) centre (6.9004, 13.23) ccw
  line L2700 (6.9004, 13.293) -> (1.0789, 13.293)
  arc A2700 (1.0789, 13.293) -> (1.0789, 13.167) centre (1.0789, 13.23) ccw
  line L2701 (8.4995, 13.167) -> (17.121, 13.167)
  arc A2701 (17.121, 13.167) -> (17.121, 13.293) centre (17.121, 13.23) ccw
  line L2702 (17.121, 13.293) -> (8.4995, 13.293)
  arc A2702 (8.4995, 13.293) -> (8.4995, 13.167) centre (8.4995, 13.23) ccw
  line L2703 (1.0789, 13.293) -> (6.7744, 13.293)
  arc A2703 (6.7744, 13.293) -> (6.7744, 13.419) centre (6.7744, 13.356) ccw
  line L2704 (6.7744, 13.419) -> (1.0789, 13.419)
  arc A2704 (1.0789, 13.419) -> (1.0789, 13.293) centre (1.0789, 13.356) ccw
  line L2705 (8.6255, 13.293) -> (17.121, 13.293)
  arc A2705 (17.121, 13.293) -> (17.121, 13.419) centre (17.121, 13.356) ccw
  line L2706 (17.121, 13.419) -> (8.6255, 13.419)
  arc A2706 (8.6255, 13.419) -> (8.6255, 13.293) centre (8.6255, 13.356) ccw
  line L2707 (1.0789, 13.419) -> (6.6484, 13.419)
  arc A2707 (6.6484, 13.419) -> (6.6484, 13.545) centre (6.6484, 13.482) ccw
  line L2708 (6.6484, 13.545) -> (1.0789, 13.545)
  arc A2708 (1.0789, 13.545) -> (1.0789, 13.419) centre (1.0789, 13.482) ccw
  line L2709 (8.7515, 13.419) -> (17.121, 13.419)
  arc A2709 (17.121, 13.419) -> (17.121, 13.545) centre (17.121, 13.482) ccw
  line L2710 (17.121, 13.545) -> (8.7515, 13.545)
  arc A2710 (8.7515, 13.545) -> (8.7515, 13.419) centre (8.7515, 13.482) ccw
  line L2711 (1.0789, 13.545) -> (6.5837, 13.545)
  arc A2711 (6.5837, 13.545) -> (6.5837, 13.671) centre (6.5837, 13.608) ccw
  line L2712 (6.5837, 13.671) -> (1.0789, 13.671)
  arc A2712 (1.0789, 13.671) -> (1.0789, 13.545) centre (1.0789, 13.608) ccw
  line L2713 (8.8161, 13.545) -> (17.121, 13.545)
  arc A2713 (17.121, 13.545) -> (17.121, 13.671) centre (17.121, 13.608) ccw
  line L2714 (17.121, 13.671) -> (8.8161, 13.671)
  arc A2714 (8.8161, 13.671) -> (8.8161, 13.545) centre (8.8161, 13.608) ccw
  line L2715 (1.0789, 13.671) -> (6.5316, 13.671)
  arc A2715 (6.5316, 13.671) -> (6.5316, 13.797) centre (6.5316, 13.734) ccw
  line L2716 (6.5316, 13.797) -> (1.0789, 13.797)
  arc A2716 (1.0789, 13.797) -> (1.0789, 13.671) centre (1.0789, 13.734) ccw
  line L2717 (8.8682, 13.671) -> (17.121, 13.671)
  arc A2717 (17.121, 13.671) -> (17.121, 13.797) centre (17.121, 13.734) ccw
  line L2718 (17.121, 13.797) -> (8.8682, 13.797)
  arc A2718 (8.8682, 13.797) -> (8.8682, 13.671) centre (8.8682, 13.734) ccw
  line L2719 (1.0789, 13.797) -> (6.4794, 13.797)
  arc A2719 (6.4794, 13.797) -> (6.4794, 13.923) centre (6.4794, 13.86) ccw
  line L2720 (6.4794, 13.923) -> (1.0789, 13.923)
  arc A2720 (1.0789, 13.923) -> (1.0789, 13.797) centre (1.0789, 13.86) ccw
  line L2721 (8.9204, 13.797) -> (17.121, 13.797)
  arc A2721 (17.121, 13.797) -> (17.121, 13.923) centre (17.121, 13.86) ccw
  line L2722 (17.121, 13.923) -> (8.9204, 13.923)
  arc A2722 (8.9204, 13.923) -> (8.9204, 13.797) centre (8.9204, 13.86) ccw
  line L2723 (1.0789, 13.923) -> (6.4346, 13.923)
  arc A2723 (6.4346, 13.923) -> (6.4346, 14.049) centre (6.4346, 13.986) ccw
  line L2724 (6.4346, 14.049) -> (1.0789, 14.049)
  arc A2724 (1.0789, 14.049) -> (1.0789, 13.923) centre (1.0789, 13.986) ccw
  line L2725 (8.9653, 13.923) -> (17.121, 13.923)
  arc A2725 (17.121, 13.923) -> (17.121, 14.049) centre (17.121, 13.986) ccw
  line L2726 (17.121, 14.049) -> (8.9653, 14.049)
  arc A2726 (8.9653, 14.049) -> (8.9653, 13.923) centre (8.9653, 13.986) ccw
  line L2727 (1.0789, 14.049) -> (6.4346, 14.049)
  arc A2727 (6.4346, 14.049) -> (6.4346, 14.175) centre (6.4346, 14.112) ccw
  line L2728 (6.4346, 14.175) -> (1.0789, 14.175)
  arc A2728 (1.0789, 14.175) -> (1.0789, 14.049) centre (1.0789, 14.112) ccw
  line L2729 (8.9653, 14.049) -> (17.121, 14.049)
  arc A2729 (17.121, 14.049) -> (17.121, 14.175) centre (17.121, 14.112) ccw
  line L2730 (17.121, 14.175) -> (8.9653, 14.175)
  arc A2730 (8.9653, 14.175) -> (8.9653, 14.049) centre (8.9653, 14.112) ccw
  line L2731 (1.0789, 14.175) -> (6.4346, 14.175)
  arc A2731 (6.4346, 14.175) -> (6.4346, 14.301) centre (6.4346, 14.238) ccw
  line L2732 (6.4346, 14.301) -> (1.0789, 14.301)
  arc A2732 (1.0789, 14.301) -> (1.0789, 14.175) centre (1.0789, 14.238) ccw
  line L2733 (8.9653, 14.175) -> (17.121, 14.175)
  arc A2733 (17.121, 14.175) -> (17.121, 14.301) centre (17.121, 14.238) ccw
  line L2734 (17.121, 14.301) -> (8.9653, 14.301)
  arc A2734 (8.9653, 14.301) -> (8.9653, 14.175) centre (8.9653, 14.238) ccw
  line L2735 (1.0789, 14.301) -> (6.4346, 14.301)
  arc A2735 (6.4346, 14.301) -> (6.4346, 14.427) centre (6.4346, 14.364) ccw
  line L2736 (6.4346, 14.427) -> (1.0789, 14.427)
  arc A2736 (1.0789, 14.427) -> (1.0789, 14.301) centre (1.0789, 14.364) ccw
  line L2737 (8.9653, 14.301) -> (17.121, 14.301)
  arc A2737 (17.121, 14.301) -> (17.121, 14.427) centre (17.121, 14.364) ccw
  line L2738 (17.121, 14.427) -> (8.9653, 14.427)
  arc A2738 (8.9653, 14.427) -> (8.9653, 14.301) centre (8.9653, 14.364) ccw
  line L2739 (1.0789, 14.427) -> (6.4422, 14.427)
  arc A2739 (6.4422, 14.427) -> (6.4422, 14.553) centre (6.4422, 14.49) ccw
  line L2740 (6.4422, 14.553) -> (1.0789, 14.553)
  arc A2740 (1.0789, 14.553) -> (1.0789, 14.427) centre (1.0789, 14.49) ccw
  line L2741 (8.9578, 14.427) -> (17.121, 14.427)
  arc A2741 (17.121, 14.427) -> (17.121, 14.553) centre (17.121, 14.49) ccw
  line L2742 (17.121, 14.553) -> (8.9578, 14.553)
  arc A2742 (8.9578, 14.553) -> (8.9578, 14.427) centre (8.9578, 14.49) ccw
  line L2743 (1.0789, 14.553) -> (6.4944, 14.553)
  arc A2743 (6.4944, 14.553) -> (6.4944, 14.679) centre (6.4944, 14.616) ccw
  line L2744 (6.4944, 14.679) -> (1.0789, 14.679)
  arc A2744 (1.0789, 14.679) -> (1.0789, 14.553) centre (1.0789, 14.616) ccw
  line L2745 (8.9056, 14.553) -> (17.121, 14.553)
  arc A2745 (17.121, 14.553) -> (17.121, 14.679) centre (17.121, 14.616) ccw
  line L2746 (17.121, 14.679) -> (8.9056, 14.679)
  arc A2746 (8.9056, 14.679) -> (8.9056, 14.553) centre (8.9056, 14.616) ccw
  line L2747 (1.0789, 14.679) -> (6.5466, 14.679)
  arc A2747 (6.5466, 14.679) -> (6.5466, 14.805) centre (6.5466, 14.742) ccw
  line L2748 (6.5466, 14.805) -> (1.0789, 14.805)
  arc A2748 (1.0789, 14.805) -> (1.0789, 14.679) centre (1.0789, 14.742) ccw
  line L2749 (8.8534, 14.679) -> (17.121, 14.679)
  arc A2749 (17.121, 14.679) -> (17.121, 14.805) centre (17.121, 14.742) ccw
  line L2750 (17.121, 14.805) -> (8.8534, 14.805)
  arc A2750 (8.8534, 14.805) -> (8.8534, 14.679) centre (8.8534, 14.742) ccw
  line L2751 (1.0789, 14.805) -> (6.5988, 14.805)
  arc A2751 (6.5988, 14.805) -> (6.5988, 14.931) centre (6.5988, 14.868) ccw
  line L2752 (6.5988, 14.931) -> (1.0789, 14.931)
  arc A2752 (1.0789, 14.931) -> (1.0789, 14.805) centre (1.0789, 14.868) ccw
  line L2753 (8.8012, 14.805) -> (17.121, 14.805)
  arc A2753 (17.121, 14.805) -> (17.121, 14.931) centre (17.121, 14.868) ccw
  line L2754 (17.121, 14.931) -> (8.8012, 14.931)
  arc A2754 (8.8012, 14.931) -> (8.8012, 14.805) centre (8.8012, 14.868) ccw
  line L2755 (1.0789, 14.931) -> (6.6845, 14.931)
  arc A2755 (6.6845, 14.931) -> (6.6845, 15.057) centre (6.6845, 14.994) ccw
  line L2756 (6.6845, 15.057) -> (1.0789, 15.057)
  arc A2756 (1.0789, 15.057) -> (1.0789, 14.931) centre (1.0789, 14.994) ccw
  line L2757 (8.7154, 14.931) -> (17.121, 14.931)
  arc A2757 (17.121, 14.931) -> (17.121, 15.057) centre (17.121, 14.994) ccw
  line L2758 (17.121, 15.057) -> (8.7154, 15.057)
  arc A2758 (8.7154, 15.057) -> (8.7154, 14.931) centre (8.7154, 14.994) ccw
  line L2759 (1.0789, 15.057) -> (6.8105, 15.057)
  arc A2759 (6.8105, 15.057) -> (6.8105, 15.183) centre (6.8105, 15.12) ccw